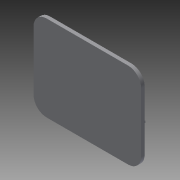
# Autodesk Inventor part: tabliczka na zasilacz
Saved by Autodesk Inventor 2014 (Build 180170000, 170)
## iProperties
Created: 2018-03-30
Part Number: tabliczka na zasilacz
Material: Generic
Document SubType Name: Modeling
Designer: HP820
Density: 1 g/cm^3
Appearance: Default
Author: HP820
Autodesk Inventor part; units mm, degrees
ref_plane "YZ Plane" through (0, 0, 0) normal (1, 0, 0) x (0, 1, 0)
ref_plane "XZ Plane" through (0, 0, 0) normal (0, 1, 0) x (-1, 0, 0)
ref_plane "XY Plane" through (0, 0, 0) normal (0, 0, 1) x (1, 0, 0)
sketch "Sketch1" plane through (0, 0, 0) normal (0, 1, 0) x (-1, 0, 0)
  line L0 (-12.3, 9.8) -> (12.3, 9.8)
  line L1 (12.3, 9.8) -> (12.3, -9.8)
  line L2 (12.3, -9.8) -> (-12.3, -9.8)
  line L3 (-12.3, -9.8) -> (-12.3, 9.8)
  line L4 (-12.3, 9.8) -> (12.3, -9.8) construction
  line L5 (12.3, 9.8) -> (-12.3, -9.8) construction
  point P0 (0, 0)
  dimension "d0" = 24.6
  dimension "d1" = 19.6
  constraints: 12 end point, 2 midpoint, 2 parallel, 1 horizontal, 1 perpendicular
  measures "d0" distance of L1.end L2.end
  measures "d1" distance of L0.end L1.end
extrude "Extrusion1" add sketch "Sketch1" along normal blind 0.8
sketch "Sketch2" plane through (0, 0.8, 0) normal (0, 1, 0) x (1, 0, 0)
  line L0 (-12.3492, 7.0634) -> (9.587, 7.0634) construction
  line L1 (9.587, 7.0634) -> (9.587, -7.3694) construction
  line L2 (9.587, -7.3694) -> (-12.3492, -7.3694) construction
  line L3 (-12.3492, -7.3694) -> (-12.3492, 7.0634) construction
  spline S0 degree 2 poles (-8.79, -0.2162) (-8.79, -0.764) (-9.2341, -1.6457) (-9.6069, -1.8921) knots 0 0 0 1 2 2 2
  spline S1 degree 2 poles (-9.6069, -1.8921) (-9.9116, -2.0833) (-10.5372, -2.213) (-11.0234, -2.213) knots 0 0 0 1 2 2 2
  line L4 (-11.0234, -2.213) -> (-11.944, -2.213)
  line L5 (-11.944, -2.213) -> (-11.944, 1.787)
  line L6 (-11.944, 1.787) -> (-11.0331, 1.787)
  spline S2 degree 2 poles (-11.0331, 1.787) (-10.4691, 1.787) (-9.8273, 1.6185) (-9.6004, 1.4694) knots 0 0 0 1 2 2 2
  spline S3 degree 2 poles (-9.6004, 1.4694) (-9.2147, 1.2133) (-8.79, 0.3673) (-8.79, -0.2162) knots 0 0 0 1 2 2 2
  spline S4 degree 2 poles (-9.3443, -0.2097) (-9.3443, 0.2506) (-9.649, 0.9021) (-9.9505, 1.0869) knots 0 0 0 1 2 2 2
  spline S5 degree 2 poles (-9.9505, 1.0869) (-10.1644, 1.2133) (-10.6474, 1.3267) (-11.0072, 1.3267) knots 0 0 0 1 2 2 2
  line L7 (-11.0072, 1.3267) -> (-11.4124, 1.3267)
  line L8 (-11.4124, 1.3267) -> (-11.4124, -1.7527)
  line L9 (-11.4124, -1.7527) -> (-11.0072, -1.7527)
  spline S6 degree 2 poles (-11.0072, -1.7527) (-10.6539, -1.7527) (-10.119, -1.6392) (-9.9018, -1.4869) knots 0 0 0 1 2 2 2
  spline S7 degree 2 poles (-9.9018, -1.4869) (-9.6231, -1.2989) (-9.3443, -0.6765) (-9.3443, -0.2097) knots 0 0 0 1 2 2 2
  spline S8 degree 2 poles (-6.9488, -2.281) (-7.6685, -2.281) (-8.4594, -1.4739) (-8.4594, -0.7284) knots 0 0 0 1 2 2 2
  spline S9 degree 2 poles (-8.4594, -0.7284) (-8.4594, 0.0042) (-7.6911, 0.8729) (-7.072, 0.8729) knots 0 0 0 1 2 2 2
  spline S10 degree 2 poles (-7.072, 0.8729) (-6.7933, 0.8729) (-6.3621, 0.7109) (-6.2033, 0.5391) knots 0 0 0 1 2 2 2
  spline S11 degree 2 poles (-6.2033, 0.5391) (-6.0412, 0.3673) (-5.8694, -0.1287) (-5.8694, -0.4885) knots 0 0 0 1 2 2 2
  line L10 (-5.8694, -0.4885) -> (-5.8694, -0.764)
  line L11 (-5.8694, -0.764) -> (-7.9472, -0.764)
  spline S12 degree 2 poles (-7.9472, -0.764) (-7.9472, -1.2859) (-7.4221, -1.8402) (-6.9553, -1.8402) knots 0 0 0 1 2 2 2
  spline S13 degree 2 poles (-6.9553, -1.8402) (-6.79, -1.8402) (-6.4691, -1.7656) (-6.3394, -1.7073) knots 0 0 0 1 2 2 2
  spline S14 degree 2 poles (-6.3394, -1.7073) (-6.2033, -1.6425) (-6.0153, -1.529) (-5.9537, -1.4772) knots 0 0 0 1 2 2 2
  line L12 (-5.9537, -1.4772) -> (-5.9245, -1.4772)
  line L13 (-5.9245, -1.4772) -> (-5.9245, -2.0282)
  spline S15 degree 2 poles (-5.9245, -2.0282) (-6.0121, -2.0639) (-6.2779, -2.1676) (-6.3816, -2.1968) knots 0 0 0 1 2 2 2
  spline S16 degree 2 poles (-6.3816, -2.1968) (-6.5275, -2.2389) (-6.7673, -2.281) (-6.9488, -2.281) knots 0 0 0 1 2 2 2
  spline S17 degree 2 poles (-6.3621, -0.3783) (-6.3686, -0.1741) (-6.4529, 0.1241) (-6.5339, 0.2246) knots 0 0 0 1 2 2 2
  spline S18 degree 2 poles (-6.5339, 0.2246) (-6.6215, 0.3381) (-6.897, 0.458) (-7.1012, 0.458) knots 0 0 0 1 2 2 2
  spline S19 degree 2 poles (-7.1012, 0.458) (-7.3022, 0.458) (-7.5842, 0.3381) (-7.7009, 0.2214) knots 0 0 0 1 2 2 2
  spline S20 degree 2 poles (-7.7009, 0.2214) (-7.8143, 0.1015) (-7.931, -0.187) (-7.9472, -0.3783) knots 0 0 0 1 2 2 2
  line L14 (-7.9472, -0.3783) -> (-6.3621, -0.3783)
  spline S21 degree 2 poles (-3.6847, -1.8953) (-3.7463, -1.9407) (-3.9537, -2.1028) (-4.051, -2.1514) knots 0 0 0 1 2 2 2
  spline S22 degree 2 poles (-4.051, -2.1514) (-4.1839, -2.2227) (-4.4335, -2.2973) (-4.6604, -2.2973) knots 0 0 0 1 2 2 2
  spline S23 degree 2 poles (-4.6604, -2.2973) (-4.8451, -2.2973) (-5.179, -2.1579) (-5.3054, -2.0314) knots 0 0 0 1 2 2 2
  spline S24 degree 2 poles (-5.3054, -2.0314) (-5.4253, -1.9083) (-5.5712, -1.5452) (-5.5712, -1.3443) knots 0 0 0 1 2 2 2
  spline S25 degree 2 poles (-5.5712, -1.3443) (-5.5712, -1.0331) (-5.3087, -0.5922) (-5.0234, -0.4658) knots 0 0 0 1 2 2 2
  spline S26 degree 2 poles (-5.0234, -0.4658) (-4.7706, -0.3491) (-4.0834, -0.2616) (-3.6847, -0.2389) knots 0 0 0 1 2 2 2
  line L15 (-3.6847, -0.2389) -> (-3.6847, -0.1417)
  spline S27 degree 2 poles (-3.6847, -0.1417) (-3.6847, 0.0334) (-3.7916, 0.2506) (-3.8889, 0.3121) knots 0 0 0 1 2 2 2
  spline S28 degree 2 poles (-3.8889, 0.3121) (-3.9861, 0.3737) (-4.2649, 0.4126) (-4.414, 0.4126) knots 0 0 0 1 2 2 2
  spline S29 degree 2 poles (-4.414, 0.4126) (-4.589, 0.4126) (-5.0623, 0.3089) (-5.2989, 0.2084) knots 0 0 0 1 2 2 2
  line L16 (-5.2989, 0.2084) -> (-5.3281, 0.2084)
  line L17 (-5.3281, 0.2084) -> (-5.3281, 0.7238)
  spline S30 degree 2 poles (-5.3281, 0.7238) (-5.1887, 0.7627) (-4.6668, 0.86) (-4.4108, 0.86) knots 0 0 0 1 2 2 2
  spline S31 degree 2 poles (-4.4108, 0.86) (-4.0996, 0.86) (-3.6749, 0.7627) (-3.5064, 0.6363) knots 0 0 0 1 2 2 2
  spline S32 degree 2 poles (-3.5064, 0.6363) (-3.3411, 0.5131) (-3.179, 0.1209) (-3.179, -0.1611) knots 0 0 0 1 2 2 2
  line L18 (-3.179, -0.1611) -> (-3.179, -2.213)
  line L19 (-3.179, -2.213) -> (-3.6847, -2.213)
  line L20 (-3.6847, -2.213) -> (-3.6847, -1.8953)
  line L21 (-3.6847, -1.4739) -> (-3.6847, -0.6408)
  spline S33 degree 2 poles (-3.6847, -0.6408) (-3.8662, -0.6571) (-4.414, -0.7122) (-4.5858, -0.764) knots 0 0 0 1 2 2 2
  spline S34 degree 2 poles (-4.5858, -0.764) (-4.7868, -0.8256) (-5.0493, -1.0817) (-5.0493, -1.3086) knots 0 0 0 1 2 2 2
  spline S35 degree 2 poles (-5.0493, -1.3086) (-5.0493, -1.5679) (-4.7576, -1.8305) (-4.4788, -1.8305) knots 0 0 0 1 2 2 2
  spline S36 degree 2 poles (-4.4788, -1.8305) (-4.2422, -1.8305) (-3.8532, -1.6263) (-3.6847, -1.4739) knots 0 0 0 1 2 2 2
  line L22 (-0.8905, 1.4791) -> (-0.9164, 1.4791)
  spline S37 degree 2 poles (-0.9164, 1.4791) (-0.9845, 1.505) (-1.2373, 1.5504) (-1.3378, 1.5504) knots 0 0 0 1 2 2 2
  spline S38 degree 2 poles (-1.3378, 1.5504) (-1.6555, 1.5504) (-1.9278, 1.2651) (-1.9278, 0.8891) knots 0 0 0 1 2 2 2
  line L23 (-1.9278, 0.8891) -> (-1.9278, 0.7886)
  line L24 (-1.9278, 0.7886) -> (-1.0915, 0.7886)
  line L25 (-1.0915, 0.7886) -> (-1.0915, 0.3705)
  line L26 (-1.0915, 0.3705) -> (-1.9116, 0.3705)
  line L27 (-1.9116, 0.3705) -> (-1.9116, -2.213)
  line L28 (-1.9116, -2.213) -> (-2.4172, -2.213)
  line L29 (-2.4172, -2.213) -> (-2.4172, 0.3705)
  line L30 (-2.4172, 0.3705) -> (-2.7576, 0.3705)
  line L31 (-2.7576, 0.3705) -> (-2.7576, 0.7886)
  line L32 (-2.7576, 0.7886) -> (-2.4172, 0.7886)
  line L33 (-2.4172, 0.7886) -> (-2.4172, 0.8891)
  spline S39 degree 2 poles (-2.4172, 0.8891) (-2.4172, 1.4272) (-1.8954, 1.9912) (-1.4091, 1.9912) knots 0 0 0 1 2 2 2
  spline S40 degree 2 poles (-1.4091, 1.9912) (-1.2698, 1.9912) (-1.0007, 1.9621) (-0.8905, 1.9426) knots 0 0 0 1 2 2 2
  line L34 (-0.8905, 1.9426) -> (-0.8905, 1.4791)
  line L35 (-1.1109, -2.213) -> (0.2375, 1.787)
  line L36 (0.2375, 1.787) -> (0.8923, 1.787)
  line L37 (0.8923, 1.787) -> (2.2408, -2.213)
  line L38 (2.2408, -2.213) -> (1.68, -2.213)
  line L39 (1.68, -2.213) -> (1.317, -1.0947)
  line L40 (1.317, -1.0947) -> (-0.2098, -1.0947)
  line L41 (-0.2098, -1.0947) -> (-0.5728, -2.213)
  line L42 (-0.5728, -2.213) -> (-1.1109, -2.213)
  line L43 (1.1711, -0.6408) -> (0.552, 1.2425)
  line L44 (0.552, 1.2425) -> (-0.0639, -0.6408)
  line L45 (-0.0639, -0.6408) -> (1.1711, -0.6408)
  line L46 (3.0965, -2.213) -> (2.5909, -2.213)
  line L47 (2.5909, -2.213) -> (2.5909, 1.9653)
  line L48 (2.5909, 1.9653) -> (3.0965, 1.9653)
  line L49 (3.0965, 1.9653) -> (3.0965, -2.213)
  spline S41 degree 2 poles (7.0317, -0.2162) (7.0317, -0.764) (6.5876, -1.6457) (6.2148, -1.8921) knots 0 0 0 1 2 2 2
  spline S42 degree 2 poles (6.2148, -1.8921) (5.9101, -2.0833) (5.2845, -2.213) (4.7983, -2.213) knots 0 0 0 1 2 2 2
  line L50 (4.7983, -2.213) -> (3.8777, -2.213)
  line L51 (3.8777, -2.213) -> (3.8777, 1.787)
  line L52 (3.8777, 1.787) -> (4.7886, 1.787)
  spline S43 degree 2 poles (4.7886, 1.787) (5.3526, 1.787) (5.9944, 1.6185) (6.2213, 1.4694) knots 0 0 0 1 2 2 2
  spline S44 degree 2 poles (6.2213, 1.4694) (6.6071, 1.2133) (7.0317, 0.3673) (7.0317, -0.2162) knots 0 0 0 1 2 2 2
  spline S45 degree 2 poles (6.4774, -0.2097) (6.4774, 0.2506) (6.1727, 0.9021) (5.8712, 1.0869) knots 0 0 0 1 2 2 2
  spline S46 degree 2 poles (5.8712, 1.0869) (5.6573, 1.2133) (5.1743, 1.3267) (4.8145, 1.3267) knots 0 0 0 1 2 2 2
  line L53 (4.8145, 1.3267) -> (4.4093, 1.3267)
  line L54 (4.4093, 1.3267) -> (4.4093, -1.7527)
  line L55 (4.4093, -1.7527) -> (4.8145, -1.7527)
  spline S47 degree 2 poles (4.8145, -1.7527) (5.1678, -1.7527) (5.7027, -1.6392) (5.9199, -1.4869) knots 0 0 0 1 2 2 2
  spline S48 degree 2 poles (5.9199, -1.4869) (6.1986, -1.2989) (6.4774, -0.6765) (6.4774, -0.2097) knots 0 0 0 1 2 2 2
  spline S49 degree 2 poles (8.8729, -2.281) (8.1533, -2.281) (7.3623, -1.4739) (7.3623, -0.7284) knots 0 0 0 1 2 2 2
  spline S50 degree 2 poles (7.3623, -0.7284) (7.3623, 0.0042) (8.1306, 0.8729) (8.7497, 0.8729) knots 0 0 0 1 2 2 2
  spline S51 degree 2 poles (8.7497, 0.8729) (9.0285, 0.8729) (9.4596, 0.7109) (9.6184, 0.5391) knots 0 0 0 1 2 2 2
  spline S52 degree 2 poles (9.6184, 0.5391) (9.7805, 0.3673) (9.9523, -0.1287) (9.9523, -0.4885) knots 0 0 0 1 2 2 2
  line L56 (9.9523, -0.4885) -> (9.9523, -0.764)
  line L57 (9.9523, -0.764) -> (7.8745, -0.764)
  spline S53 degree 2 poles (7.8745, -0.764) (7.8745, -1.2859) (8.3996, -1.8402) (8.8664, -1.8402) knots 0 0 0 1 2 2 2
  spline S54 degree 2 poles (8.8664, -1.8402) (9.0317, -1.8402) (9.3526, -1.7656) (9.4823, -1.7073) knots 0 0 0 1 2 2 2
  spline S55 degree 2 poles (9.4823, -1.7073) (9.6184, -1.6425) (9.8064, -1.529) (9.868, -1.4772) knots 0 0 0 1 2 2 2
  line L58 (9.868, -1.4772) -> (9.8972, -1.4772)
  line L59 (9.8972, -1.4772) -> (9.8972, -2.0282)
  spline S56 degree 2 poles (9.8972, -2.0282) (9.8097, -2.0639) (9.5439, -2.1676) (9.4401, -2.1968) knots 0 0 0 1 2 2 2
  spline S57 degree 2 poles (9.4401, -2.1968) (9.2943, -2.2389) (9.0544, -2.281) (8.8729, -2.281) knots 0 0 0 1 2 2 2
  spline S58 degree 2 poles (9.4596, -0.3783) (9.4531, -0.1741) (9.3688, 0.1241) (9.2878, 0.2246) knots 0 0 0 1 2 2 2
  spline S59 degree 2 poles (9.2878, 0.2246) (9.2003, 0.3381) (8.9247, 0.458) (8.7205, 0.458) knots 0 0 0 1 2 2 2
  spline S60 degree 2 poles (8.7205, 0.458) (8.5195, 0.458) (8.2375, 0.3381) (8.1208, 0.2214) knots 0 0 0 1 2 2 2
  spline S61 degree 2 poles (8.1208, 0.2214) (8.0074, 0.1015) (7.8907, -0.187) (7.8745, -0.3783) knots 0 0 0 1 2 2 2
  line L60 (7.8745, -0.3783) -> (9.4596, -0.3783)
  line L61 (12.056, 0.2473) -> (12.0301, 0.2473)
  spline S62 degree 2 poles (12.0301, 0.2473) (11.9717, 0.2635) (11.8453, 0.27) (11.7578, 0.27) knots 0 0 0 1 2 2 2
  spline S63 degree 2 poles (11.7578, 0.27) (11.5536, 0.27) (11.1516, 0.0917) (10.9701, -0.0833) knots 0 0 0 1 2 2 2
  line L62 (10.9701, -0.0833) -> (10.9701, -2.213)
  line L63 (10.9701, -2.213) -> (10.4644, -2.213)
  line L64 (10.4644, -2.213) -> (10.4644, 0.7886)
  line L65 (10.4644, 0.7886) -> (10.9701, 0.7886)
  line L66 (10.9701, 0.7886) -> (10.9701, 0.3413)
  spline S64 degree 2 poles (10.9701, 0.3413) (11.2456, 0.5877) (11.6573, 0.7886) (11.8518, 0.7886) knots 0 0 0 1 2 2 2
  spline S65 degree 2 poles (11.8518, 0.7886) (11.9296, 0.7886) (12.0074, 0.7822) (12.056, 0.7724) knots 0 0 0 1 2 2 2
  line L67 (12.056, 0.7724) -> (12.056, 0.2473)
  point P0 (0, 0)
  constraints: 2 other
extrude "Extrusion2" add sketch "Sketch2" along normal blind 0.4
fillet "Fillet1" radius 3 4 edges at (12.3, 0.4, 9.8) (12.3, 0.4, -9.8) (-12.3, 0.4, -9.8) (-12.3, 0.4, 9.8)
body "Solid1"
